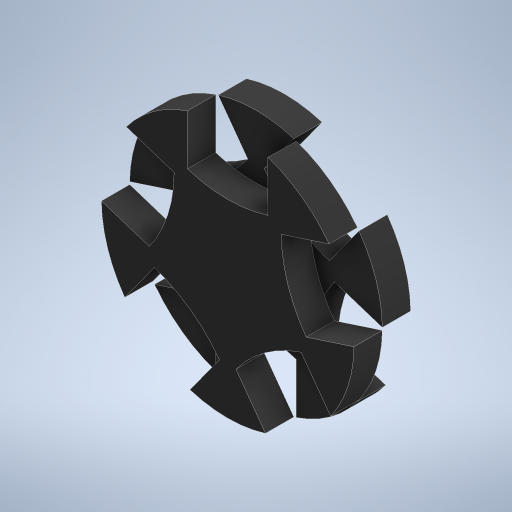
# Autodesk Inventor part: base
Saved by Autodesk Inventor 2024.1 (Build 281209000, 209)
## iProperties
Created: 2024-11-26
Part Number: base
Material: ゴム
Document SubType Name: Modeling
Designer: hibik
Density: 0.93 g/cm^3
Appearance: ゴム - 黒
Author: hibik
Autodesk Inventor part; units mm, degrees
ref_plane "YZ Plane" through (0, 0, 0) normal (1, 0, 0) x (0, 1, 0)
ref_plane "XZ Plane" through (0, 0, 0) normal (0, 1, 0) x (-1, 0, 0)
ref_plane "XY Plane" through (0, 0, 0) normal (0, 0, 1) x (1, 0, 0)
sketch "スケッチ1" plane through (0, 0, 0) normal (0, 0, 1) x (1, 0, 0)
  circle A0 centre (0, 0) radius 29
  line L0 (-9.25, 29) -> (9.25, 29)
  line L1 (9.25, 29) -> (9.25, 0)
  line L2 (9.25, 0) -> (-9.25, 0)
  line L3 (-9.25, 0) -> (-9.25, 29)
  line L4 (-9.25, 22.5) -> (9.25, 22.5)
  arc A1 (-9.25, 17.5148) -> (9.25, 17.5148) centre (0, 45) ccw
  arc A2 (-9.25, 15.9365) -> (9.25, 15.9365) centre (0, 45) ccw
  point P0 (9.25, 27.4852)
  point P1 (-9.25, 27.4852)
  point P2 (0, 22.5)
  point P3 (0, 22.5)
  dimension "d0" = 58
  dimension "d1" = 18.5
  dimension "d2" = 6.5
  dimension "d9" = 1.5
  constraints: 10 end point, 6 point on line, 4 midpoint, 4 point on circle, 3 centre point, 2 coincident, 2 parallel, 2 perpendicular, 2 vertical alignment, 1 concentric, 1 horizontal, 1 tangent, 1 other
  measures "d0" diameter of A0
  measures "d1" distance of L0.start L0.end
  measures "d2" distance between parallel lines of L0 L4
  measures "d9" radial gap between concentric circles of A1 A2
extrude "押し出し3" add sketch "スケッチ1" along normal blind 6.5 contours A0 L3 L2 L1 | L1 L4 L3 A0 | L1 A1 L3 L4 | L1 A2 L3 A1 | L1 L2 L3 A2
extrude "押し出し4" cut sketch "スケッチ1" along normal blind 6.5 contours L1 L4 L3 A0 | L1 A1 L3 L4 | L1 A2 L3 A1
pattern_circular "円形状パターン1" count 5 over 360 about axis through (0, 0, -10) along (0, 0, 1) of "押し出し4"
sketch "スケッチ4" plane through (0, 0, 0) normal (0, 0, -1) x (-1, 0, 0)
  arc A0 (-9.25, 27.4852) -> (-23.2816, 17.2907) centre (0, 0) ccw projected
  circle A1 centre (0, 0) radius 29
  line L0 (-9.25, 15.9365) -> (-9.25, 27.4852) construction
  arc A2 (-9.25, 15.9365) -> (9.25, 15.9365) centre (0, 45) ccw construction
  line L1 (9.25, 27.4852) -> (9.25, 15.9365) construction
  line L2 (40.6, 0) -> (-40.6, 0) construction
  line L3 (-9.25, -15.9365) -> (-9.25, -27.4852)
  arc A3 (9.25, -15.9365) -> (-9.25, -15.9365) centre (0, -45) ccw
  line L4 (9.25, -27.4852) -> (9.25, -15.9365)
  point P0 (-9.25, 27.4852)
  point P1 (-23.2816, 17.2907)
  constraints: 5 symmetric about line, 4 end point, 2 point on circle, 1 centre point, 1 coincident, 4 other
extrude "押し出し5" add sketch "スケッチ4" along normal blind 6.5
extrude "押し出し6" cut sketch "スケッチ4" along normal blind 6.5 contours L3 A3 L4 A1
pattern_circular "円形状パターン2" count 5 over 360 about axis through (0, 0, -10) along (0, 0, 1) of "押し出し6"
